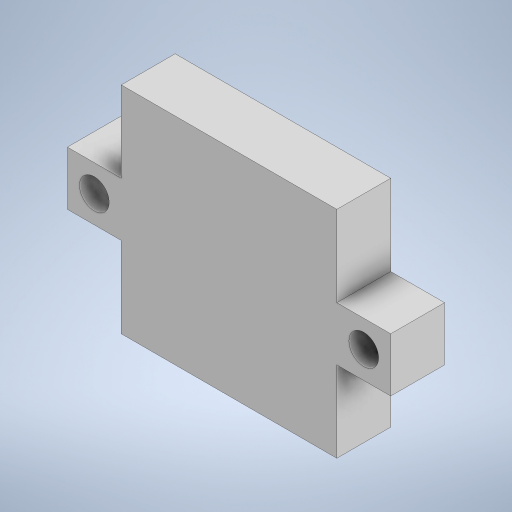
# Autodesk Inventor part: cap5V
Saved by Autodesk Inventor 2023 (Build 270158000, 158)
## iProperties
Created: 2023-05-22
Part Number: cap5V
Material: 一般
Document SubType Name: Modeling
Designer: 310611102
Density: 1 g/cm^3
Appearance: 預設
Author: 310611102
Autodesk Inventor part; units mm, degrees
ref_plane "YZ Plane" through (0, 0, 0) normal (1, 0, 0) x (0, 1, 0)
ref_plane "XZ Plane" through (0, 0, 0) normal (0, 1, 0) x (-1, 0, 0)
ref_plane "XY Plane" through (0, 0, 0) normal (0, 0, 1) x (1, 0, 0)
sketch "Sketch1" plane through (0, 0, 0) normal (0, 0, 1) x (1, 0, 0)
  line L0 (-20, 20) -> (20, 20)
  line L1 (20, 20) -> (20, -20)
  line L2 (20, -20) -> (-20, -20)
  line L3 (-20, -20) -> (-20, 20)
  line L4 (-20, 20) -> (20, -20) construction
  line L5 (20, 20) -> (-20, -20) construction
  line L6 (20, -5) -> (30, -5)
  line L7 (30, -5) -> (30, 5)
  line L8 (30, 5) -> (20, 5)
  line L9 (20, 5) -> (20, -5)
  line L10 (-20, -5) -> (-30, -5)
  line L11 (-30, -5) -> (-30, 5)
  line L12 (-30, 5) -> (-20, 5)
  line L13 (-20, 5) -> (-20, -5)
  circle A0 centre (-25, 0) radius 2.75
  circle A1 centre (25, 0) radius 2.75
  point P0 (0, 0)
  point P1 (30, 0)
  point P2 (20, 0)
  point P3 (-25, 5)
  point P4 (25, 5)
  dimension "d0" = 40
  dimension "d1" = 40
  dimension "d2" = 10
  dimension "d3" = 10
  dimension "d4" = 10
  dimension "d5" = 5.5
  dimension "d6" = 5.5
  constraints: 28 end point, 6 midpoint, 6 parallel, 4 point on line, 3 horizontal, 3 horizontal alignment, 3 perpendicular, 2 centre point, 2 vertical alignment
  measures "d0" distance of L0.start L0.end
  measures "d1" distance of L0.end L1.end
  measures "d2" distance of L6.end L7.end
  measures "d3" distance of L7.end L8.end
  measures "d4" distance of L11.end L12.end
  measures "d5" diameter of A1
  measures "d6" diameter of A0
extrude "Extrusion1" add sketch "Sketch1" along normal blind 10
body "Solid1"
